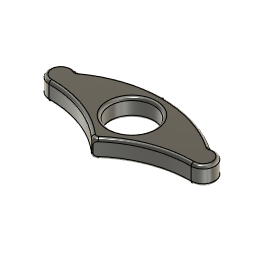
Book (Autodesk Fusion 360 design; units mm, degrees)
Autodesk Fusion 360 part; units mm, degrees
note: some values were not read from the file. Set by a fixed rule: which face or edge a step refers to.
sketch "Sketch1" plane through (0, 0, 0) normal (0, 0, 1) x (1, 0, 0)
  circle A0 centre (0, 0) radius 12
  circle A1 centre (0, 0) radius 17.5
  circle A2 centre (-39, 0) radius 6.5
  circle A3 centre (39, 0) radius 6.5
  line L0 (0, 0) -> (0, -22)
  arc A4 (0, -22) -> (-38.9676, -6.4999) centre (-38.6884, -62.5308) ccw
  arc A5 (38.9676, -6.4999) -> (0, -22) centre (38.6884, -62.5308) ccw
  arc A6 (0, 17.5) -> (-35.8235, 5.6709) centre (0, -42.659) ccw
  arc A7 (36.7233, 6.0883) -> (0, 17.5) centre (0, -47.2943) ccw
  dimension "d1" = 24
  dimension "d2" = 35
  dimension "d5" = 13
  dimension "d6" = 39
  dimension "d7" = 22
  constraint coincident A0.centre A1.centre
  constraint equal A2 A3
  constraint vertical L0
  constraint symmetric A2.centre A3.centre L0
  constraint horizontal A0.centre A2.centre
  constraint tangent A1 A4
  constraint coincident A2 A4.end
  constraint tangent A1 A5
  constraint coincident A3 A5.start
  constraint coincident A2 A6.end
  constraint coincident A1 A6.start
  constraint coincident A3 A7.start
  constraint tangent A1 A6
  constraint tangent A1 A7
  constraint tangent A3 A5
  constraint tangent A2 A4
  constraint vertical A0.centre A6.start
  measures "d1" diameter of A0
  measures "d2" diameter of A1
  measures "d5" diameter of A2
  measures "d6" horizontal distance of A0.centre A2.centre
  measures "d7" distance of A0.centre L0.end A1.centre
extrude "Extrude1" add sketch "Sketch1" along normal blind 10
fillet "Fillet1" radius 1.5 2 faces at (21.8024, 1.0931, 10) (21.8024, 1.0931, 0)
fillet "Fillet1" radius 0.5 5 faces at (8.1139, -15.5762, 3.3333) (45.4926, -0.3103, 6.6667) (37.3356, 6.2833, 6.6667) (-8.1139, -15.5762, 6.6667) (-40.5377, -6.3155, 6.6667)
